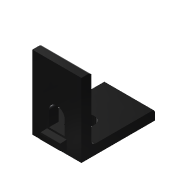
# Autodesk Inventor part: HBLFSR5_b
Saved by Autodesk Inventor 2020.1 (Build 241239000, 239)
## iProperties
Created: 2019-06-06
Part Number: HBLFSR5_b
Material: Acetal Resin, Black
Catalog Web Link: www.cadenas.de
Description: HBLFSR5_body-Tabbed Brackets -Nut Mounting Brackets-
Vendor: MISUMI
Document SubType Name: Modeling
Designer: psadmin
Manufacturer: MISUMI
Mass: 3.10733 g
Surface Area: 17.2616 cm^2
Volume: 2.18059 cm^3
Density: 1.425 g/cm^3
Appearance: Smooth - Black
Category: PARTsolutions
Company: MISUMI
PSOL_IDENT_0: {$CADENAS_DATA\23d-libs\misumi\metric\38_al_extrusions_blackets\5\hblfsr5\hblfsr5_body.prj},171 {VTY
PSOL_IDENT_1: P=3D},{NB=HBLFSR5_b},{LINA=HBLFSR5},{NN=HBLFSR5_body},{DATE=30.03.2018 06:53:34},{GEOMDATE=04.04.201
PSOL_IDENT_2: 7 02:54:30},{VERSION=},{LINEID=10},{WBVAR=ALT1,ALT2},{WBNUMERIC=}  {NB=HBLFSR5_b},{LINA=HBLFSR5},{KT=
PSOL_IDENT_3: DUMMY},{PN=HBLFSR5},{TYPE=HBLFSR5},{ALT1=},{ALT2=}
NN: HBLFSR5_body
NT: Tabbed Brackets -Nut Mounting Brackets-
NB: HBLFSR5_b
NBSYN: $PN._b
LINA: HBLFSR5
PN: HBLFSR5
TYPE: HBLFSR5
ALT1: w/o C (Mounting Holes for Cover)
ALT2: w/o (Set Applicable Bolt and Nut)
SUPPLIER: MISUMI
ARTICLENO: HBLFSR5_b
BOMINFO: HBLFSR5
CREATOR: CADENAS GmbH
Title: HBLFSR5
Author: Cadenas PARTsolutions
Comments: Tabbed Brackets -Nut Mounting Brackets-
Autodesk Inventor part; units mm, degrees
ref_plane "YZ Plane" through (0, 0, 0) normal (1, 0, 0) x (0, 1, 0)
ref_plane "XZ Plane" through (0, 0, 0) normal (0, 1, 0) x (-1, 0, 0)
sketch "_____1" plane through (0, 0, 0) normal (1, 0, 0) x (0, 0, -1)
  line L0 (-30, 2.6786) -> (-30, 0)
  line L1 (-30, 0) -> (0, 0)
  line L2 (0, 0) -> (0, 30)
  line L3 (0, 30) -> (-2.6786, 30)
  arc A0 (-2.6786, 30) -> (-3.815, 29.5293) centre (-2.6786, 28.3929) ccw
  line L4 (-3.815, 29.5293) -> (-29.5293, 3.815)
  arc A1 (-29.5293, 3.815) -> (-30, 2.6786) centre (-28.3929, 2.6786) ccw
  dimension "d42" = 30
  constraints: 10 end point, 4 point on circle, 2 centre point, 1 coincident
  measures "d42" distance of L0.end L1.end
extrude "Extrusion1" add sketch "_____1" along normal mid plane 20
sketch "_____2" plane through (0, 0, 0) normal (1, 0, 0) x (0, 0, -1)
  line L0 (-32, 32) -> (-32, 4)
  line L1 (-32, 4) -> (-6, 4)
  arc A0 (-6, 4) -> (-4, 6) centre (-6, 6) ccw
  line L2 (-4, 6) -> (-4, 32)
  line L3 (-4, 32) -> (-32, 32)
  constraints: 8 end point, 2 point on circle, 1 centre point
extrude "Extrusion2" cut sketch "_____2" along normal mid plane 30
sketch "_____9" plane through (0, 0, 0) normal (1, 0, 0) x (0, 0, -1)
  line L0 (0, 5) -> (0, 1.8718)
  line L1 (0, 1.8718) -> (1.592, 2.2984)
  arc A0 (1.592, 2.2984) -> (2, 2.7898) centre (1.5, 2.7898) ccw
  line L2 (2, 2.7898) -> (2, 4.7898)
  arc A1 (2, 4.7898) -> (1.9797, 4.9309) centre (1.5, 4.7898) ccw
  line L3 (1.9797, 4.9309) -> (0, 5)
  line L4 (-30, 0) -> (0, 0) projected
  line L5 (0, 0) -> (0, 30) projected
  dimension "d34" = 0.5
  dimension "d35" = 0.5
  dimension "d36" = 15
  dimension "d37" = 2
  dimension "d38" = 2
  dimension "d40" = 2
  dimension "d41" = 5
  constraints: 8 end point, 4 point on circle, 2 centre point, 2 tangent, 1 collinear
  measures "d34" radius of A0
  measures "d35" radius of A1
  measures "d36" angle of L4 L1
  measures "d37" angle of L4 L3
  measures "d38" distance between parallel lines of L5 L2
  measures "d40" distance of A0.centre A1.centre
  measures "d41" distance of L4.end L0.start
extrude "Extrusion3" add sketch "_____9" along normal mid plane 8
sketch "_____10" plane through (0, 0, 0) normal (1, 0, 0) x (0, 0, -1)
  line L0 (-5.2401, 0) -> (-5.1188, -2.524)
  arc A0 (-5.1188, -2.524) -> (-4.6194, -3) centre (-4.6194, -2.5) ccw
  line L1 (-4.6194, -3) -> (-3.0897, -3)
  arc A1 (-3.0897, -3) -> (-2.6413, -2.7213) centre (-3.0897, -2.5) ccw
  line L2 (-2.6413, -2.7213) -> (-1.298, 0)
  line L3 (-1.298, 0) -> (-5.2401, 0)
  line L4 (0, 0) -> (-30, 0) projected
  line L5 (0, 30) -> (0, 0) projected
  dimension "d26" = 0.5
  dimension "d27" = 0.5
  dimension "d28" = 3
  dimension "d29" = 2.749
  constraints: 8 end point, 4 point on circle, 4 tangent, 2 centre point, 1 collinear
  measures "d26" radius of A0
  measures "d27" radius of A1
  measures "d28" distance between parallel lines of L3 L1
  measures "d29" angle of L5 L0
extrude "Extrusion4" add sketch "_____10" along normal mid plane 8
sketch "_____3" plane through (0, 0, 0) normal (0, 1, 0) x (1, 0, 0)
  arc A0 (-3.2, -12) -> (3.2, -12) centre (0, -12) ccw
  line L0 (3.2, -12) -> (3.2, -6)
  line L1 (3.2, -6) -> (-3.2, -6)
  line L2 (-3.2, -6) -> (-3.2, -12)
  line L3 (-10, 0) -> (10, 0) projected
  line L4 (0, -6) -> (0, 0) construction
  point P0 (-3.2, -9)
  point P1 (3.2, -9)
  dimension "d23" = 3.2
  dimension "d24" = 6
  dimension "d25" = 6
  constraints: 8 end point, 4 midpoint, 3 vertical, 2 point on circle, 1 centre point, 1 parallel, 1 tangent
  measures "d23" radius of A0
  measures "d24" distance between parallel lines of L3 L1
  measures "d25" distance from line of A0.centre L1
extrude "Extrusion5" cut sketch "_____3" along normal blind 4
ref_plane "Work Plane7" through (-10, 4, 4) normal (0, 0.7071, -0.7071) x (-1, 0, 0)
mirror "Mirror1" about plane through (-10, 4, 4) normal (0, 0.7071, -0.7071) of "Extrusion5"
body "Solid1"
